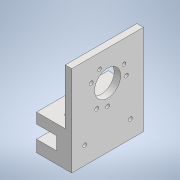
# Autodesk Inventor part: enc holder
Saved by Autodesk Inventor 2022 (Build 260153000, 153)
## iProperties
Created: 2022-05-06
Part Number: enc holder
Material: Generic
Document SubType Name: Modeling
Designer: erasm
Density: 1 g/cm^3
Appearance: Default
Author: erasm
Autodesk Inventor part; units mm, degrees
ref_plane "YZ Plane" through (0, 0, 0) normal (1, 0, 0) x (0, 1, 0)
ref_plane "XZ Plane" through (0, 0, 0) normal (0, 1, 0) x (-1, 0, 0)
ref_plane "XY Plane" through (0, 0, 0) normal (0, 0, 1) x (1, 0, 0)
sketch "Sketch1" plane through (0, 0, 0) normal (0, 0, 1) x (1, 0, 0)
  line L0 (10, 10) -> (-10, 10) construction
  line L1 (-10, 10) -> (-10, -10) construction
  line L2 (-10, -10) -> (10, -10) construction
  line L3 (10, -10) -> (10, 10) construction
  line L4 (-7, -7) -> (-7, 7) construction
  line L5 (-7, 7) -> (7, 7) construction
  line L6 (7, 7) -> (7, -7) construction
  line L7 (7, -7) -> (-7, -7) construction
  line L8 (10, 10) -> (-10, 10)
  line L9 (-10, 10) -> (-10, -10)
  line L10 (-10, -10) -> (10, -10)
  line L11 (10, -10) -> (10, 10)
  line L12 (13, 13) -> (-13, 13)
  line L13 (-13, 13) -> (-13, -13)
  line L14 (-13, -13) -> (13, -13)
  line L15 (13, -13) -> (13, 13)
  point P0 (0, 0)
  dimension "d1" = 3
  dimension "d2" = 3
  dimension "d3" = 3
  dimension "d4" = 3
  constraints: 16 end point, 4 parallel, 2 horizontal, 2 perpendicular
  measures "d1" distance between parallel lines of L0 L12
  measures "d2" distance between parallel lines of L15 L3
  measures "d3" distance between parallel lines of L14 L10
  measures "d4" distance between parallel lines of L13 L1
extrude "Extrusion1" add sketch "Sketch1" against normal blind 55
sketch "Sketch2" plane through (-13, -13, 0) normal (-1, 0, 0) x (0, 0, 1)
  line L0 (-80.4804, 18) -> (40.5, 18)
  line L1 (40.5, 18) -> (40.5, 8)
  line L2 (40.5, 8) -> (-80.4804, 8)
  line L3 (-80.4804, 8) -> (-80.4804, 18)
  line L4 (0, 26) -> (-55, 26) projected
  point P0 (0, 13)
  dimension "d7" = 10
  dimension "d8" = 8
  constraints: 8 end point, 2 parallel, 1 horizontal, 1 perpendicular
  measures "d7" distance between parallel lines of L2 L0
  measures "d8" distance between parallel lines of L4 L0
extrude "Extrusion2" cut sketch "Sketch2" against normal blind 15.3125
sketch "Sketch3" plane through (-13, 13, 0) normal (0, 1, 0) x (1, 0, 0)
  line L0 (26, 0) -> (0, 0) projected
  line L1 (3, 55) -> (23, 55) projected
  line L2 (26, 0) -> (21, 0)
  line L3 (21, 0) -> (21, 55)
  line L4 (21, 55) -> (26, 55)
  line L5 (26, 55) -> (26, 0)
  point P0 (13, 0)
  dimension "d11" = 5
  constraints: 8 end point, 2 parallel, 1 horizontal, 1 perpendicular, 1 point on line
  measures "d11" distance of L3.end L4.end
extrude "Extrusion3" add sketch "Sketch3" along normal blind 42.3
sketch "Sketch4" plane through (13, -13, 0) normal (1, 0, 0) x (0, 0, -1)
  line L0 (0, 26) -> (55, 26) projected
  circle A0 centre (27.5, 45) radius 18
  line L1 (0, 68.3) -> (55, 68.3) projected
  circle A1 centre (27.5, 45) radius 3
  point P0 (0, 13)
  point P1 (27.5, 68.3)
  dimension "d14" = 36
  dimension "d15" = 19
  dimension "d16" = 6
  constraints: 2 centre point, 1 coincident, 1 midpoint, 1 vertical alignment
  measures "d14" diameter of A0
  measures "d15" distance from line of L0 A0.centre
  measures "d16" diameter of A1
extrude "Extrusion4" cut sketch "Sketch4" against normal blind 42.3 contours A1
sketch "Sketch5" plane through (13, -13, 0) normal (1, 0, 0) x (0, 0, -1)
  circle A0 centre (27.5, 45) radius 3 projected
  circle A1 centre (27.5, 45) radius 10
  point P0 (0, 13)
  dimension "d19" = 20
  constraints: 1 centre point, 1 coincident
  measures "d19" diameter of A1
extrude "Extrusion5" cut sketch "Sketch5" against normal blind 42.3
sketch "Sketch6" plane through (13, -13, 0) normal (1, 0, 0) x (0, 0, -1)
  circle A0 centre (27.5, 30.5) radius 1.5 projected
  circle A1 centre (19.1831, 33.1223) radius 1.495 projected
  circle A2 centre (14.9426, 52.25) radius 1.5 projected
  circle A3 centre (21.372, 58.1415) radius 1.495 projected
  circle A4 centre (40.0574, 52.25) radius 1.5 projected
  circle A5 centre (41.9448, 43.7362) radius 1.495 projected
  point P0 (0, 13)
extrude "Extrusion6" cut sketch "Sketch6" against normal blind 42.3
sketch "Sketch7" plane through (13, -13, 0) normal (1, 0, 0) x (0, 0, -1)
  circle A0 centre (10, 13) radius 1.5
  circle A1 centre (45, 13) radius 1.5
  line L0 (0, 0) -> (0, 68.3) projected
  line L1 (55, 0) -> (55, 68.3) projected
  point P0 (0, 13)
  dimension "d24" = 3
  dimension "d25" = 3
  dimension "d26" = 10
  dimension "d27" = 10
  constraints: 2 centre point, 2 horizontal alignment
  measures "d24" diameter of A0
  measures "d25" diameter of A1
  measures "d26" distance from line of L0 A0.centre
  measures "d27" distance from line of L1 A1.centre
extrude "Extrusion7" cut sketch "Sketch7" against normal blind 10
sketch "Sketch8" plane through (-13, -13, 0) normal (0, -1, 0) x (1, 0, 0)
  circle A0 centre (13, -10) radius 1.5
  circle A1 centre (13, -45) radius 1.5
  line L0 (26, -55) -> (0, -55) projected
  line L1 (0, 0) -> (26, 0) projected
  point P0 (13, 0)
  point P1 (13, 0)
  point P2 (13, 0)
  dimension "d30" = 3
  dimension "d31" = 3
  dimension "d32" = 10
  dimension "d33" = 10
  constraints: 2 centre point, 2 midpoint, 2 vertical alignment
  measures "d30" diameter of A0
  measures "d31" diameter of A1
  measures "d32" distance from line of L0 A1.centre
  measures "d33" distance from line of L1 A0.centre
extrude "Extrusion8" cut sketch "Sketch8" against normal through all
body "Solid1"
